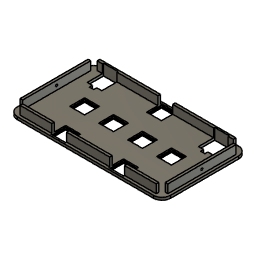
Case Top (14.4mm Switch Holes) (Autodesk Fusion 360 design; units mm, degrees)
Autodesk Fusion 360 part; units mm, degrees
sketch "Top" plane through (0, 0, 0) normal (0, 1, 0) x (1, 0, 0)
  line L0 (-80, 50) -> (80, 50)
  line L1 (90, 40) -> (90, -40)
  line L2 (80, -50) -> (-80, -50)
  line L3 (-90, -40) -> (-90, 40)
  line L4 (-90, 50) -> (90, -50) construction
  line L5 (90, 50) -> (-90, -50) construction
  arc A0 (-80, 50) -> (-90, 40) centre (-80, 40) ccw
  arc A1 (90, 40) -> (80, 50) centre (80, 40) ccw
  arc A2 (80, -50) -> (90, -40) centre (80, -40) ccw
  arc A3 (-90, -40) -> (-80, -50) centre (-80, -40) ccw
  dimension "d310" = 180
  dimension "d311" = 100
  dimension "d312" = 10
  constraint horizontal L0
  constraint perpendicular L0 L1
  constraint parallel L0 L2
  constraint parallel L1 L3
  constraint coincident L4 origin
  constraint coincident L5 origin
  constraint coincident L4.start L3
  constraint coincident L4.start L0
  constraint tangent L3 A0
  constraint tangent L0 A0
  constraint coincident L5.start L0
  constraint coincident L5.start L1
  constraint tangent L0 A1
  constraint tangent L1 A1
  constraint equal A0 A1
  constraint coincident L4.end L2
  constraint coincident L4.end L1
  constraint tangent L2 A2
  constraint tangent L1 A2
  constraint equal A0 A2
  constraint coincident L5.end L2
  constraint coincident L5.end L3
  constraint tangent L2 A3
  constraint tangent L3 A3
  constraint equal A0 A3
  measures "d310" distance of L4.end L5.end
  measures "d311" distance of L5.start L4.end
  measures "d312" radius of A0
extrude "Extrude37" add sketch "Top" along normal blind 3
sketch "Tabs" plane through (0, 3, 0) normal (0, 1, 0) x (-1, 0, 0)
  arc A0 (80, -50) -> (90, -40) centre (80, -40) ccw
  line L0 (90, -40) -> (90, 40)
  arc A1 (90, 40) -> (80, 50) centre (80, 40) ccw
  line L1 (80, 50) -> (-80, 50)
  arc A2 (-80, 50) -> (-90, 40) centre (-80, 40) ccw
  line L2 (-90, 40) -> (-90, -40)
  arc A3 (-90, -40) -> (-80, -50) centre (-80, -40) ccw
  line L3 (-80, -50) -> (80, -50)
  line L4 (86.8, -40) -> (83.8, -40)
  line L5 (83.8, -40) -> (83.8, 40)
  line L6 (83.8, 40) -> (86.8, 40)
  line L7 (86.8, 40) -> (86.8, -40)
  line L8 (86.8, -40) -> (83.8, 40) construction
  line L9 (83.8, -40) -> (86.8, 40) construction
  line L10 (80, -46.8) -> (-80, -46.8)
  line L11 (-80, -46.8) -> (-80, -43.8)
  line L12 (-80, -43.8) -> (80, -43.8)
  line L13 (80, -43.8) -> (80, -46.8)
  line L14 (80, -46.8) -> (-80, -43.8) construction
  line L15 (-80, -46.8) -> (80, -43.8) construction
  line L16 (80, 43.8) -> (-80, 43.8)
  line L17 (-80, 43.8) -> (-80, 46.8)
  line L18 (-80, 46.8) -> (80, 46.8)
  line L19 (80, 46.8) -> (80, 43.8)
  line L20 (80, 43.8) -> (-80, 46.8) construction
  line L21 (-80, 43.8) -> (80, 46.8) construction
  line L22 (-83.8, -40) -> (-86.8, -40)
  line L23 (-86.8, -40) -> (-86.8, 40)
  line L24 (-86.8, 40) -> (-83.8, 40)
  line L25 (-83.8, 40) -> (-83.8, -40)
  line L26 (-83.8, -40) -> (-86.8, 40) construction
  line L27 (-86.8, -40) -> (-83.8, 40) construction
  point P0 (85.3, 0)
  point P1 (0, -45.3)
  point P2 (0, 45.3)
  point P3 (-85.3, 0)
  dimension "d315" = 3
  dimension "d316" = 10
  dimension "d317" = 10
  dimension "d318" = 3.2
  dimension "d319" = 3
  dimension "d320" = 10
  dimension "d321" = 10
  dimension "d322" = 3.2
  dimension "d324" = 3
  dimension "d325" = 10
  dimension "d326" = 10
  dimension "d327" = 3
  dimension "d329" = 10
  dimension "d330" = 10
  dimension "d333" = 3.2
  dimension "d334" = 3.2
  constraint horizontal L4
  constraint perpendicular L4 L5
  constraint parallel L4 L6
  constraint parallel L5 L7
  constraint coincident L8 P0
  constraint coincident L9 P0
  constraint horizontal L10
  constraint perpendicular L10 L11
  constraint parallel L10 L12
  constraint parallel L11 L13
  constraint coincident L14 P1
  constraint coincident L15 P1
  constraint horizontal L16
  constraint perpendicular L16 L17
  constraint parallel L16 L18
  constraint parallel L17 L19
  constraint coincident L20 P2
  constraint coincident L21 P2
  constraint horizontal L22
  constraint perpendicular L22 L23
  constraint parallel L22 L24
  constraint parallel L23 L25
  constraint coincident L26 P3
  constraint coincident L27 P3
  measures "d315" distance of L5.end L6.end
  measures "d316" distance of L3 L4
  measures "d317" distance of L1 L6
  measures "d318" distance of L0 L7
  measures "d319" distance of L10.end L11.end
  measures "d320" distance of L0 L13
  measures "d321" distance of L2 L11
  measures "d322" distance of L3 L10
  measures "d324" distance of L16.end L17.end
  measures "d325" distance of L0 L19
  measures "d326" distance of L2 L17
  measures "d327" distance of L23.end L24.end
  measures "d329" distance of L3 L22
  measures "d330" distance of L1 L24
  measures "d333" distance of L1 L18
  measures "d334" distance of L2 L23
extrude "Extrude38" add sketch "Tabs" along normal blind 10 contours L4 L5 L6 L7 | L10 L11 L12 L13 | L16 L17 L18 L19 | L22 L23 L24 L25
sketch "Switches" plane through (0, 3, 0) normal (0, 1, 0) x (-1, 0, 0)
  line L0 (86.8, 40) -> (86.8, -40)
  line L1 (86.8, -40) -> (83.8, -40)
  line L2 (83.8, -40) -> (83.8, 40)
  line L3 (83.8, 40) -> (86.8, 40)
  line L4 (80, -43.8) -> (80, -46.8)
  line L5 (80, -46.8) -> (-80, -46.8)
  line L6 (-80, -46.8) -> (-80, -43.8)
  line L7 (-80, -43.8) -> (80, -43.8)
  line L8 (80, 46.8) -> (80, 43.8)
  line L9 (80, 43.8) -> (-80, 43.8)
  line L10 (-80, 43.8) -> (-80, 46.8)
  line L11 (-80, 46.8) -> (80, 46.8)
  line L12 (-83.8, 40) -> (-83.8, -40)
  line L13 (-83.8, -40) -> (-86.8, -40)
  line L14 (-86.8, -40) -> (-86.8, 40)
  line L15 (-86.8, 40) -> (-83.8, 40)
  arc A0 (80, -50) -> (90, -40) centre (80, -40) ccw
  line L16 (90, -40) -> (90, 40)
  arc A1 (90, 40) -> (80, 50) centre (80, 40) ccw
  line L17 (80, 50) -> (-80, 50)
  arc A2 (-80, 50) -> (-90, 40) centre (-80, 40) ccw
  line L18 (-90, 40) -> (-90, -40)
  arc A3 (-90, -40) -> (-80, -50) centre (-80, -40) ccw
  line L19 (-80, -50) -> (80, -50)
  line L20 (-59.7, 8.7) -> (-42.3, 8.7)
  line L21 (-42.3, 8.7) -> (-42.3, -8.7)
  line L22 (-58.2, -7.2) -> (-58.2, 7.2)
  line L23 (-42.3, -8.7) -> (-59.7, -8.7)
  line L24 (-43.8, 7.2) -> (-43.8, -7.2)
  line L25 (-58.2, 7.2) -> (-43.8, 7.2)
  line L26 (-43.8, -7.2) -> (-58.2, 7.2) construction
  line L27 (-59.7, -8.7) -> (-59.7, 8.7)
  line L28 (-59.7, -8.7) -> (-42.3, 8.7) construction
  line L29 (-58.2, -7.2) -> (-43.8, 7.2) construction
  line L30 (-42.3, -8.7) -> (-59.7, 8.7) construction
  line L31 (-43.8, -7.2) -> (-58.2, -7.2)
  line L32 (24.2, 7.2) -> (24.2, -7.2)
  line L33 (8.3, -8.7) -> (8.3, 8.7)
  line L34 (25.7, -8.7) -> (8.3, 8.7) construction
  line L35 (9.8, 7.2) -> (24.2, 7.2)
  line L36 (24.2, -7.2) -> (9.8, 7.2) construction
  line L37 (8.3, -8.7) -> (25.7, 8.7) construction
  line L38 (9.8, -7.2) -> (24.2, 7.2) construction
  line L39 (24.2, -7.2) -> (9.8, -7.2)
  line L40 (25.7, 8.7) -> (25.7, -8.7)
  line L41 (9.8, -7.2) -> (9.8, 7.2)
  line L42 (25.7, -8.7) -> (8.3, -8.7)
  line L43 (8.3, 8.7) -> (25.7, 8.7)
  line L44 (-26.8, 32.1) -> (-41.2, 46.5) construction
  line L45 (-41.2, 46.5) -> (-26.8, 46.5)
  line L46 (-25.3, 30.6) -> (-42.7, 30.6)
  line L47 (-42.7, 48) -> (-25.3, 48)
  line L48 (-41.2, 32.1) -> (-41.2, 46.5)
  line L49 (-25.3, 48) -> (-25.3, 30.6)
  line L50 (-42.7, 30.6) -> (-42.7, 48)
  line L51 (-25.3, 30.6) -> (-42.7, 48) construction
  line L52 (-26.8, 32.1) -> (-41.2, 32.1)
  line L53 (-41.2, 32.1) -> (-26.8, 46.5) construction
  line L54 (-42.7, 30.6) -> (-25.3, 48) construction
  line L55 (-26.8, 46.5) -> (-26.8, 32.1)
  line L56 (25.3, 30.6) -> (42.7, 48) construction
  line L57 (26.8, 46.5) -> (41.2, 46.5)
  line L58 (42.7, 48) -> (42.7, 30.6)
  line L59 (26.8, 32.1) -> (41.2, 46.5) construction
  line L60 (41.2, 32.1) -> (26.8, 32.1)
  line L61 (25.3, 30.6) -> (25.3, 48)
  line L62 (41.2, 46.5) -> (41.2, 32.1)
  line L63 (25.3, 48) -> (42.7, 48)
  line L64 (42.7, 30.6) -> (25.3, 48) construction
  line L65 (42.7, 30.6) -> (25.3, 30.6)
  line L66 (26.8, 32.1) -> (26.8, 46.5)
  line L67 (41.2, 32.1) -> (26.8, 46.5) construction
  line L68 (-8.7, -48) -> (-8.7, -30.6)
  line L69 (-7.2, -46.5) -> (-7.2, -32.1)
  line L70 (7.2, -32.1) -> (7.2, -46.5)
  line L71 (-7.2, -46.5) -> (7.2, -32.1) construction
  line L72 (8.7, -30.6) -> (8.7, -48)
  line L73 (8.7, -48) -> (-8.7, -48)
  line L74 (7.2, -46.5) -> (-7.2, -32.1) construction
  line L75 (8.7, -48) -> (-8.7, -30.6) construction
  line L76 (-8.7, -48) -> (8.7, -30.6) construction
  line L77 (-8.7, -30.6) -> (8.7, -30.6)
  line L78 (7.2, -46.5) -> (-7.2, -46.5)
  line L79 (-7.2, -32.1) -> (7.2, -32.1)
  line L80 (42.3, -8.7) -> (42.3, 8.7)
  line L81 (43.8, 7.2) -> (58.2, 7.2)
  line L82 (42.3, 8.7) -> (59.7, 8.7)
  line L83 (59.7, -8.7) -> (42.3, -8.7)
  line L84 (58.2, -7.2) -> (43.8, -7.2)
  line L85 (58.2, 7.2) -> (58.2, -7.2)
  line L86 (42.3, -8.7) -> (59.7, 8.7) construction
  line L87 (59.7, -8.7) -> (42.3, 8.7) construction
  line L88 (43.8, -7.2) -> (43.8, 7.2)
  line L89 (43.8, -7.2) -> (58.2, 7.2) construction
  line L90 (58.2, -7.2) -> (43.8, 7.2) construction
  line L91 (59.7, 8.7) -> (59.7, -8.7)
  line L92 (-25.7, 8.7) -> (-8.3, 8.7)
  line L93 (-25.7, -8.7) -> (-8.3, 8.7) construction
  line L94 (-25.7, -8.7) -> (-25.7, 8.7)
  line L95 (-9.8, 7.2) -> (-9.8, -7.2)
  line L96 (-9.8, -7.2) -> (-24.2, -7.2)
  line L97 (-8.3, -8.7) -> (-25.7, 8.7) construction
  line L98 (-24.2, -7.2) -> (-9.8, 7.2) construction
  line L99 (-8.3, -8.7) -> (-25.7, -8.7)
  line L100 (-24.2, -7.2) -> (-24.2, 7.2)
  line L101 (-9.8, -7.2) -> (-24.2, 7.2) construction
  line L102 (-8.3, 8.7) -> (-8.3, -8.7)
  line L103 (-24.2, 7.2) -> (-9.8, 7.2)
  line L104 (80, 50) -> (-80, 50)
  point P0 (-51, 0)
  point P1 (17, 0)
  point P2 (-34, 39.3)
  point P3 (34, 39.3)
  point P4 (0, -39.3)
  point P5 (51, 0)
  point P6 (-17, 0)
  dimension "d345" = 14.4
  dimension "d346" = 14.4
  dimension "d347" = 1.5
  dimension "d348" = 1.5
  dimension "d349" = 1.5
  dimension "d350" = 1.5
  dimension "d363" = 14.4
  dimension "d364" = 14.4
  dimension "d365" = 1.5
  dimension "d366" = 1.5
  dimension "d367" = 1.5
  dimension "d368" = 1.5
  dimension "d369" = 14.4
  dimension "d370" = 14.4
  dimension "d371" = 1.5
  dimension "d372" = 1.5
  dimension "d373" = 1.5
  dimension "d374" = 1.5
  dimension "d375" = 14.4
  dimension "d376" = 14.4
  dimension "d377" = 1.5
  dimension "d378" = 1.5
  dimension "d379" = 1.5
  dimension "d380" = 1.5
  dimension "d381" = 14.4
  dimension "d382" = 14.4
  dimension "d383" = 1.5
  dimension "d384" = 1.5
  dimension "d385" = 1.5
  dimension "d386" = 1.5
  dimension "d387" = 14.4
  dimension "d388" = 14.4
  dimension "d389" = 1.5
  dimension "d390" = 1.5
  dimension "d391" = 1.5
  dimension "d392" = 1.5
  dimension "d393" = 14.4
  dimension "d394" = 14.4
  dimension "d395" = 1.5
  dimension "d396" = 1.5
  dimension "d397" = 1.5
  dimension "d398" = 1.5
  dimension "d406" = 34
  dimension "d407" = 34
  dimension "d408" = 34
  dimension "d409" = 17
  dimension "d445" = 2
  dimension "d446" = 2
  dimension "d447" = 2
  dimension "d459" = 17
  dimension "d460" = 17
  constraint horizontal L31
  constraint perpendicular L22 L31
  constraint parallel L25 L31
  constraint parallel L22 L24
  constraint coincident P0 L26
  constraint coincident P0 L29
  constraint horizontal L23
  constraint perpendicular L23 L27
  constraint parallel L20 L23
  constraint parallel L21 L27
  constraint horizontal L39
  constraint perpendicular L39 L41
  constraint parallel L35 L39
  constraint parallel L32 L41
  constraint coincident P1 L36
  constraint coincident P1 L38
  constraint horizontal L42
  constraint perpendicular L33 L42
  constraint parallel L42 L43
  constraint parallel L33 L40
  constraint horizontal L52
  constraint perpendicular L48 L52
  constraint parallel L45 L52
  constraint parallel L48 L55
  constraint coincident P2 L44
  constraint coincident P2 L53
  constraint horizontal L46
  constraint perpendicular L46 L50
  constraint parallel L46 L47
  constraint parallel L49 L50
  constraint horizontal L60
  constraint perpendicular L60 L66
  constraint parallel L57 L60
  constraint parallel L62 L66
  constraint coincident P3 L67
  constraint coincident P3 L59
  constraint horizontal L65
  constraint perpendicular L61 L65
  constraint parallel L63 L65
  constraint parallel L58 L61
  constraint horizontal L78
  constraint perpendicular L69 L78
  constraint parallel L78 L79
  constraint parallel L69 L70
  constraint coincident P4 L74
  constraint coincident P4 L71
  constraint horizontal L73
  constraint perpendicular L68 L73
  constraint parallel L73 L77
  constraint parallel L68 L72
  constraint vertical origin P4
  constraint horizontal origin P1
  constraint horizontal origin P0
  constraint horizontal L84
  constraint perpendicular L84 L88
  constraint parallel L81 L84
  constraint parallel L85 L88
  constraint coincident P5 L90
  constraint coincident P5 L89
  constraint horizontal L83
  constraint perpendicular L80 L83
  constraint parallel L82 L83
  constraint parallel L80 L91
  constraint horizontal L96
  constraint perpendicular L96 L100
  constraint parallel L96 L103
  constraint parallel L95 L100
  constraint coincident P6 L101
  constraint coincident P6 L98
  constraint horizontal L99
  constraint perpendicular L94 L99
  constraint parallel L92 L99
  constraint parallel L94 L102
  constraint horizontal origin P6
  constraint horizontal origin P5
  measures "d345" distance of L22.end L24.start
  measures "d346" distance of L22.start L22.end
  measures "d347" distance of L23 L31
  measures "d348" distance of L21 L24
  measures "d349" distance of L20 L25
  measures "d350" distance of L22 L27
  measures "d363" distance of L35.start L32.start
  measures "d364" distance of L38.start L35.start
  measures "d365" distance of L39 L42
  measures "d366" distance of L32 L40
  measures "d367" distance of L35 L43
  measures "d368" distance of L33 L41
  measures "d369" distance of L45.end L44.end
  measures "d370" distance of L48.start L44.end
  measures "d371" distance of L46 L52
  measures "d372" distance of L49 L55
  measures "d373" distance of L45 L47
  measures "d374" distance of L48 L50
  measures "d375" distance of L57.start L57.end
  measures "d376" distance of L59.start L57.start
  measures "d377" distance of L60 L65
  measures "d378" distance of L58 L62
  measures "d379" distance of L57 L63
  measures "d380" distance of L61 L66
  measures "d381" distance of L70.start L69.end
  measures "d382" distance of L69.start L69.end
  measures "d383" distance of L73 L78
  measures "d384" distance of L70 L72
  measures "d385" distance of L77 L79
  measures "d386" distance of L68 L69
  measures "d387" distance of L81.end L81.start
  measures "d388" distance of L84.end L81.start
  measures "d389" distance of L83 L84
  measures "d390" distance of L85 L91
  measures "d391" distance of L81 L82
  measures "d392" distance of L80 L88
  measures "d393" distance of L100.end L95.start
  measures "d394" distance of L100.end L96.end
  measures "d395" distance of L96 L99
  measures "d396" distance of L95 L102
  measures "d397" distance of L92 L103
  measures "d398" distance of L94 L100
  measures "d406" distance of P1 P5
  measures "d407" distance of P1 P6
  measures "d408" distance of P0 P6
  measures "d409" distance of origin P1
  measures "d445" distance of L19 L73
  measures "d446" distance of L47 L104
  measures "d447" distance of L63 L104
  measures "d459" horizontal distance of P3 P5
  measures "d460" horizontal distance of P0 P2
extrude "Extrude40" cut sketch "Switches" against normal blind 1.7 contours L5 L7 L68 L69 L70 L72 L78 | L7 L68 L69 L70 L72 L77 L79 | L5 L68 L72 L73 | L9 L11 L57 L58 L61 L62 L66 | L11 L58 L61 L63 | L9 L58 L60 L61 L62 L65 L66 | L9 L11 L45 L48 L49 L50 L55 | L11 L47 L49 L50 | L9 L46 L48 L49 L50 L52 L55 | L20 L21 L23 L27 | L33 L40 L42 L43 | L80 L82 L83 L91 | L92 L94 L99 L102
extrude "Extrude41" cut sketch "Switches" along normal blind 3 from surface at -3 contours L7 L69 L70 L78 | L7 L69 L70 L79 | L9 L60 L62 L66 | L9 L57 L62 L66 | L9 L48 L52 L55 | L9 L45 L48 L55 | L22 L24 L25 L31 | L32 L35 L39 L41 | L81 L84 L85 L88 | L95 L96 L100 L103
sketch "Tab Holes" plane through (0, 0, 0) normal (1, 0, 0) x (0, 0, -1)
  circle A0 centre (0, 8) radius 1.25
  line L0 (-40, 3) -> (40, 3)
  dimension "d418" = 2.5
  dimension "d419" = 5
  measures "d418" diameter of A0
  measures "d419" distance of A0.centre L0
extrude "Extrude42" cut sketch "Tab Holes" along normal through all and the other way through all
sketch "Encoders" plane through (0, 3, 0) normal (0, 1, 0) x (-1, 0, 0)
  line L0 (73.8, -26) -> (56.8, -26)
  line L1 (56.8, -26) -> (56.8, -45)
  line L2 (56.8, -45) -> (73.8, -45)
  line L3 (73.8, -45) -> (73.8, -26)
  line L4 (73.8, -26) -> (56.8, -45) construction
  line L5 (56.8, -26) -> (73.8, -45) construction
  line L6 (67.8, -26) -> (62.8, -26)
  line L7 (62.8, -26) -> (62.8, -22.5)
  line L8 (62.8, -22.5) -> (67.8, -22.5)
  line L9 (67.8, -22.5) -> (67.8, -26)
  arc A0 (80, -50) -> (90, -40) centre (80, -40) ccw
  line L10 (90, -40) -> (90, 40)
  arc A1 (90, 40) -> (80, 50) centre (80, 40) ccw
  line L11 (80, 50) -> (-80, 50)
  arc A2 (-80, 50) -> (-90, 40) centre (-80, 40) ccw
  line L12 (-90, 40) -> (-90, -40)
  arc A3 (-90, -40) -> (-80, -50) centre (-80, -40) ccw
  line L13 (-80, -50) -> (80, -50)
  line L14 (-83.8, 40) -> (-83.8, -40)
  line L15 (-83.8, -40) -> (-86.8, -40)
  line L16 (-86.8, -40) -> (-86.8, 40)
  line L17 (-86.8, 40) -> (-83.8, 40)
  line L18 (80, 46.8) -> (80, 43.8)
  line L19 (80, 43.8) -> (42.7, 43.8)
  line L20 (-80, 43.8) -> (-80, 46.8)
  line L21 (-25.3, 46.8) -> (25.3, 46.8)
  line L22 (80, -43.8) -> (80, -46.8)
  line L23 (-8.7, -46.8) -> (-80, -46.8)
  line L24 (-80, -46.8) -> (-80, -43.8)
  line L25 (-80, -43.8) -> (-8.7, -43.8)
  line L26 (86.8, 40) -> (86.8, -40)
  line L27 (86.8, -40) -> (83.8, -40)
  line L28 (83.8, -40) -> (83.8, 40)
  line L29 (83.8, 40) -> (86.8, 40)
  line L30 (25.3, 48) -> (42.7, 48)
  line L31 (42.7, 48) -> (42.7, 46.8)
  line L32 (42.7, 30.6) -> (25.3, 30.6)
  line L33 (25.3, 46.8) -> (25.3, 48)
  line L34 (8.7, -48) -> (-8.7, -48)
  line L35 (-8.7, -48) -> (-8.7, -46.8)
  line L36 (-8.7, -30.6) -> (8.7, -30.6)
  line L37 (8.7, -30.6) -> (8.7, -43.8)
  line L38 (25.7, -8.7) -> (8.3, -8.7)
  line L39 (8.3, -8.7) -> (8.3, 8.7)
  line L40 (8.3, 8.7) -> (25.7, 8.7)
  line L41 (25.7, 8.7) -> (25.7, -8.7)
  line L42 (-25.3, 48) -> (-25.3, 46.8)
  line L43 (-25.3, 30.6) -> (-42.7, 30.6)
  line L44 (-42.7, 46.8) -> (-42.7, 48)
  line L45 (-42.7, 48) -> (-25.3, 48)
  line L46 (-25.7, -8.7) -> (-25.7, 8.7)
  line L47 (-25.7, 8.7) -> (-8.3, 8.7)
  line L48 (-8.3, 8.7) -> (-8.3, -8.7)
  line L49 (-8.3, -8.7) -> (-25.7, -8.7)
  line L50 (42.3, -8.7) -> (42.3, 8.7)
  line L51 (42.3, 8.7) -> (59.7, 8.7)
  line L52 (59.7, 8.7) -> (59.7, -8.7)
  line L53 (59.7, -8.7) -> (42.3, -8.7)
  line L54 (-42.3, 8.7) -> (-42.3, -8.7)
  line L55 (-42.3, -8.7) -> (-59.7, -8.7)
  line L56 (-59.7, -8.7) -> (-59.7, 8.7)
  line L57 (-59.7, 8.7) -> (-42.3, 8.7)
  line L58 (-56.8, -26) -> (-73.8, -26)
  line L59 (-67.8, -22.5) -> (-62.8, -22.5)
  line L60 (-73.8, -45) -> (-56.8, -45)
  line L61 (-67.8, -26) -> (-67.8, -22.5)
  line L62 (-73.8, -26) -> (-73.8, -45)
  line L63 (-62.8, -22.5) -> (-62.8, -26)
  line L64 (-56.8, -26) -> (-73.8, -45) construction
  line L65 (-73.8, -26) -> (-56.8, -45) construction
  line L66 (-56.8, -45) -> (-56.8, -26)
  line L67 (-62.8, -26) -> (-67.8, -26)
  line L68 (42.7, 46.8) -> (80, 46.8)
  line L69 (42.7, 43.8) -> (42.7, 30.6)
  line L70 (25.3, 30.6) -> (25.3, 43.8)
  line L71 (25.3, 43.8) -> (-25.3, 43.8)
  line L72 (-25.3, 43.8) -> (-25.3, 30.6)
  line L73 (-42.7, 30.6) -> (-42.7, 43.8)
  line L74 (-42.7, 43.8) -> (-80, 43.8)
  line L75 (-80, 46.8) -> (-42.7, 46.8)
  line L76 (-8.7, -43.8) -> (-8.7, -30.6)
  line L77 (8.7, -43.8) -> (80, -43.8)
  line L78 (80, -46.8) -> (8.7, -46.8)
  line L79 (8.7, -46.8) -> (8.7, -48)
  point P0 (65.3, -35.5)
  point P1 (-65.3, -35.5)
  dimension "d421" = 17
  dimension "d422" = 19
  dimension "d423" = 5
  dimension "d424" = 3.5
  dimension "d425" = 2.5
  dimension "d431" = 17
  dimension "d432" = 19
  dimension "d433" = 5
  dimension "d434" = 3.5
  dimension "d435" = 2.5
  dimension "d437" = 10
  dimension "d439" = 10
  dimension "d443" = 5
  dimension "d444" = 5
  constraint horizontal L0
  constraint perpendicular L0 L1
  constraint parallel L0 L2
  constraint parallel L1 L3
  constraint coincident L4 P0
  constraint coincident L5 P0
  constraint horizontal L6
  constraint vertical L7
  constraint horizontal L8
  constraint vertical L9
  constraint coincident L0 L6.start
  constraint horizontal L58
  constraint perpendicular L58 L62
  constraint parallel L58 L60
  constraint parallel L62 L66
  constraint coincident P1 L64
  constraint coincident P1 L65
  constraint horizontal L67
  constraint vertical L61
  constraint horizontal L59
  constraint vertical L63
  constraint coincident L63.end L58
  measures "d421" distance of L1.end L2.end
  measures "d422" distance of L0.end L1.end
  measures "d423" distance of L6.start L6.end
  measures "d424" distance of L6.start L8.end
  measures "d425" distance of P0 L9
  measures "d431" distance of L60.start L60.end
  measures "d432" distance of L58.end L60.start
  measures "d433" distance of L61.start L63.end
  measures "d434" distance of L59.end L63.end
  measures "d435" distance of P1 L63
  measures "d437" distance of L3 L28
  measures "d439" distance of L14 L62
  measures "d443" distance of L13 L60
  measures "d444" distance of L2 L13
extrude "Extrude43" cut sketch "Encoders" along normal blind 3 from surface at -3 contours L0 L1 L3 L6 L77 | L0 L6 L7 L8 L9 | L1 L2 L3 L77
extrude "Extrude44" cut sketch "Encoders" along normal blind 3 from surface at -3 contours L25 L60 L62 L66 | L25 L58 L62 L66 L67 | L58 L59 L61 L63 L67
extrude "Extrude45" cut sketch "Encoders" along normal through all contours L25 L60 L62 L66
extrude "Extrude46" cut sketch "Encoders" along normal through all contours L1 L2 L3 L77
extrude "Extrude47" cut sketch "Switches" along normal through all contours L9 L11 L45 L48 L49 L50 L55 | L9 L45 L48 L55
extrude "Extrude48" cut sketch "Switches" along normal through all contours L9 L11 L57 L58 L61 L62 L66 | L9 L57 L62 L66
extrude "Extrude49" cut sketch "Switches" along normal through all contours L5 L7 L68 L69 L70 L72 L78 | L7 L69 L70 L78
equation "d409 = ( 34 / 2 ) * 1 mm"
equation "d413 = -( 3 mm - 1.3 mm )"
equation "d419 = ( 10 / 2 ) * 1 mm"
equation "d425 = ( 5 / 2 ) * 1 mm"
equation "d435 = ( 5 / 2 ) * 1 mm"
equation "d459 = ( 34 / 2 ) * 1 mm"
equation "d460 = ( 34 / 2 ) * 1 mm"
named bodies: "Body"
